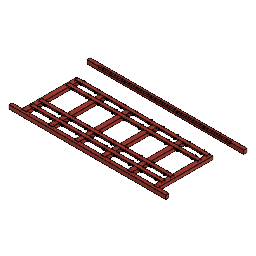
world (Autodesk Fusion 360 archive; units mm, degrees)
design "Maverick metal"
Autodesk Fusion 360 part; units mm, degrees
(part 1 of 2)
ref_plane "WorkPlane1" through (0, 0, -19.05) normal (0, 0, 1) x (1, 0, 0)
ref_plane "WorkPlane2" through (0, 0, -22.225) normal (0, 0, 1) x (1, 0, 0)
sketch "metal1" plane through (0, 0, 0) normal (0, 0, 1) x (1, 0, 0)
  circle A0 centre (67.0555, -55.245) radius 4.3815
  circle A1 centre (22.2245, -55.245) radius 4.3815
  circle A2 centre (25.2725, -93.218) radius 2.54
  circle A3 centre (64.0075, -93.218) radius 2.54
  line L0 (6.0955, -80.518) -> (-0.0005, -80.518)
  line L1 (6.0955, -96.393) -> (6.0955, -80.518)
  arc A4 (6.0955, -96.393) -> (9.2705, -99.568) centre (9.2705, -96.393) ccw
  line L2 (80.0095, -99.568) -> (9.2705, -99.568)
  arc A5 (80.0095, -99.568) -> (83.1845, -96.393) centre (80.0095, -96.393) ccw
  line L3 (83.1845, -80.518) -> (83.1845, -96.393)
  line L4 (89.2805, -80.518) -> (83.1845, -80.518)
  line L5 (89.2805, 938.276) -> (89.2805, -80.518)
  line L6 (-0.0005, 938.276) -> (89.2805, 938.276)
  line L7 (-0.0005, -80.518) -> (-0.0005, 938.276)
  circle A6 centre (2540.5075, -93.218) radius 2.54
  circle A7 centre (2543.5555, -55.245) radius 4.3815
  circle A8 centre (2498.7245, -55.245) radius 4.3815
  arc A9 (2501.7725, -95.758) -> (2501.7852, -90.678) centre (2501.7725, -93.218) ccw
  arc A10 (2501.7852, -90.678) -> (2501.7725, -95.758) centre (2501.7852, -93.218) ccw
  line L8 (2482.5955, -80.518) -> (2476.4995, -80.518)
  line L9 (2482.5955, -96.393) -> (2482.5955, -80.518)
  arc A11 (2482.5955, -96.393) -> (2485.7705, -99.568) centre (2485.7705, -96.393) ccw
  line L10 (2556.5095, -99.568) -> (2485.7705, -99.568)
  arc A12 (2556.5095, -99.568) -> (2559.6845, -96.393) centre (2556.5095, -96.393) ccw
  line L11 (2559.6845, -80.518) -> (2559.6845, -96.393)
  line L12 (2565.7805, -80.518) -> (2559.6845, -80.518)
  line L13 (2565.7805, 938.276) -> (2565.7805, -80.518)
  line L14 (2476.4995, 938.276) -> (2565.7805, 938.276)
  line L15 (2476.4995, -80.518) -> (2476.4995, 938.276)
  circle A13 centre (520.5725, -93.218) radius 2.54
  circle A14 centre (562.3555, -55.245) radius 4.3815
  circle A15 centre (517.5245, -55.245) radius 4.3815
  circle A16 centre (559.3075, -93.218) radius 2.54
  line L16 (501.3955, -80.518) -> (495.2995, -80.518)
  line L17 (501.3955, -96.393) -> (501.3955, -80.518)
  arc A17 (501.3955, -96.393) -> (504.5705, -99.568) centre (504.5705, -96.393) ccw
  line L18 (575.3095, -99.568) -> (504.5705, -99.568)
  arc A18 (575.3095, -99.568) -> (578.4845, -96.393) centre (575.3095, -96.393) ccw
  line L19 (578.4845, -80.518) -> (578.4845, -96.393)
  line L20 (584.5805, -80.518) -> (578.4845, -80.518)
  line L21 (584.5805, 938.276) -> (584.5805, -80.518)
  line L22 (495.2995, 938.276) -> (584.5805, 938.276)
  line L23 (495.2995, -80.518) -> (495.2995, 938.276)
  circle A19 centre (1549.9075, -93.218) radius 2.54
  circle A20 centre (1508.1245, -55.245) radius 4.3815
  circle A21 centre (1552.9555, -55.245) radius 4.3815
  arc A22 (1511.1852, -90.678) -> (1511.1725, -95.758) centre (1511.1852, -93.218) ccw
  arc A23 (1511.1725, -95.758) -> (1511.1852, -90.678) centre (1511.1725, -93.218) ccw
  line L24 (1491.9955, -80.518) -> (1485.8995, -80.518)
  line L25 (1491.9955, -96.393) -> (1491.9955, -80.518)
  arc A24 (1491.9955, -96.393) -> (1495.1705, -99.568) centre (1495.1705, -96.393) ccw
  line L26 (1565.9095, -99.568) -> (1495.1705, -99.568)
  arc A25 (1565.9095, -99.568) -> (1569.0845, -96.393) centre (1565.9095, -96.393) ccw
  line L27 (1569.0845, -80.518) -> (1569.0845, -96.393)
  line L28 (1575.1805, -80.518) -> (1569.0845, -80.518)
  line L29 (1575.1805, 938.276) -> (1575.1805, -80.518)
  line L30 (1485.8995, 938.276) -> (1575.1805, 938.276)
  line L31 (1485.8995, -80.518) -> (1485.8995, 938.276)
  circle A26 centre (2048.2555, -55.245) radius 4.3815
  circle A27 centre (2003.4245, -55.245) radius 4.3815
  arc A28 (2006.4725, -95.758) -> (2006.4852, -90.678) centre (2006.4725, -93.218) ccw
  arc A29 (2006.4852, -90.678) -> (2006.4725, -95.758) centre (2006.4852, -93.218) ccw
  arc A30 (2045.2075, -95.758) -> (2045.2202, -90.678) centre (2045.2075, -93.218) ccw
  arc A31 (2045.2202, -90.678) -> (2045.2075, -95.758) centre (2045.2202, -93.218) ccw
  line L32 (1987.2955, -80.518) -> (1981.1995, -80.518)
  line L33 (1987.2955, -96.393) -> (1987.2955, -80.518)
  arc A32 (1987.2955, -96.393) -> (1990.4705, -99.568) centre (1990.4705, -96.393) ccw
  line L34 (2061.2095, -99.568) -> (1990.4705, -99.568)
  arc A33 (2061.2095, -99.568) -> (2064.3845, -96.393) centre (2061.2095, -96.393) ccw
  line L35 (2064.3845, -80.518) -> (2064.3845, -96.393)
  line L36 (2070.4805, -80.518) -> (2064.3845, -80.518)
  line L37 (2070.4805, 938.276) -> (2070.4805, -80.518)
  line L38 (1981.1995, 938.276) -> (2070.4805, 938.276)
  line L39 (1981.1995, -80.518) -> (1981.1995, 938.276)
  circle A34 centre (1015.8725, -93.218) radius 2.54
  circle A35 centre (1012.8245, -55.245) radius 4.3815
  circle A36 centre (1057.6555, -55.245) radius 4.3815
  circle A37 centre (1054.6075, -93.218) radius 2.54
  line L40 (996.6955, -80.518) -> (990.5995, -80.518)
  line L41 (996.6955, -96.393) -> (996.6955, -80.518)
  arc A38 (996.6955, -96.393) -> (999.8705, -99.568) centre (999.8705, -96.393) ccw
  line L42 (1070.6095, -99.568) -> (999.8705, -99.568)
  arc A39 (1070.6095, -99.568) -> (1073.7845, -96.393) centre (1070.6095, -96.393) ccw
  line L43 (1073.7845, -80.518) -> (1073.7845, -96.393)
  line L44 (1079.8805, -80.518) -> (1073.7845, -80.518)
  line L45 (1079.8805, 938.276) -> (1079.8805, -80.518)
  line L46 (990.5995, 938.276) -> (1079.8805, 938.276)
  line L47 (990.5995, -80.518) -> (990.5995, 938.276)
sketch "metal2" plane through (0, 0, 0) normal (0, 0, 1) x (1, 0, 0)
  circle A0 centre (1690.5727, -112.268) radius 2.54
  circle A1 centre (1944.5727, -112.268) radius 2.54
  circle A2 centre (1891.2327, -112.268) radius 2.54
  circle A3 centre (621.2327, -112.268) radius 2.54
  circle A4 centre (2452.5727, -112.268) radius 2.54
  circle A5 centre (166.5727, -112.268) radius 2.54
  circle A6 centre (928.5727, -112.268) radius 2.54
  circle A7 centre (-87.4273, -112.268) radius 2.54
  circle A8 centre (1637.2327, -112.268) radius 2.54
  circle A9 centre (1436.5727, -112.268) radius 2.54
  circle A10 centre (367.2327, -112.268) radius 2.54
  circle A11 centre (1182.5727, -112.268) radius 2.54
  circle A12 centre (2145.2327, -112.268) radius 2.54
  circle A13 centre (2653.2327, -112.268) radius 2.54
  circle A14 centre (1383.2327, -112.268) radius 2.54
  circle A15 centre (420.5727, -112.268) radius 2.54
  circle A16 centre (875.2327, -112.268) radius 2.54
  circle A17 centre (2198.5727, -112.268) radius 2.54
  circle A18 centre (674.5727, -112.268) radius 2.54
  circle A19 centre (113.2327, -112.268) radius 2.54
  circle A20 centre (2399.2327, -112.268) radius 2.54
  circle A21 centre (1129.2327, -112.268) radius 2.54
  line L0 (2559.6845, -96.393) -> (2559.6845, -80.518)
  arc A22 (2556.5095, -99.568) -> (2559.6845, -96.393) centre (2556.5095, -96.393) ccw
  line L1 (2485.7705, -99.568) -> (2556.5095, -99.568)
  arc A23 (2482.5955, -96.393) -> (2485.7705, -99.568) centre (2485.7705, -96.393) ccw
  line L2 (2482.5955, -80.518) -> (2482.5955, -96.393)
  line L3 (2064.3845, -80.518) -> (2482.5955, -80.518)
  line L4 (2064.3845, -96.393) -> (2064.3845, -80.518)
  arc A24 (2061.2095, -99.568) -> (2064.3845, -96.393) centre (2061.2095, -96.393) ccw
  line L5 (1990.4705, -99.568) -> (2061.2095, -99.568)
  arc A25 (1987.2955, -96.393) -> (1990.4705, -99.568) centre (1990.4705, -96.393) ccw
  line L6 (1987.2955, -80.518) -> (1987.2955, -96.393)
  line L7 (1569.0845, -80.518) -> (1987.2955, -80.518)
  line L8 (1569.0845, -96.393) -> (1569.0845, -80.518)
  arc A26 (1565.9095, -99.568) -> (1569.0845, -96.393) centre (1565.9095, -96.393) ccw
  line L9 (1495.1705, -99.568) -> (1565.9095, -99.568)
  arc A27 (1491.9955, -96.393) -> (1495.1705, -99.568) centre (1495.1705, -96.393) ccw
  line L10 (1491.9955, -80.518) -> (1491.9955, -96.393)
  line L11 (1073.7845, -80.518) -> (1491.9955, -80.518)
  line L12 (1073.7845, -96.393) -> (1073.7845, -80.518)
  arc A28 (1070.6095, -99.568) -> (1073.7845, -96.393) centre (1070.6095, -96.393) ccw
  line L13 (999.8705, -99.568) -> (1070.6095, -99.568)
  arc A29 (996.6955, -96.393) -> (999.8705, -99.568) centre (999.8705, -96.393) ccw
  line L14 (996.6955, -80.518) -> (996.6955, -96.393)
  line L15 (578.4845, -80.518) -> (996.6955, -80.518)
  line L16 (578.4845, -96.393) -> (578.4845, -80.518)
  arc A30 (575.3095, -99.568) -> (578.4845, -96.393) centre (575.3095, -96.393) ccw
  line L17 (504.5705, -99.568) -> (575.3095, -99.568)
  arc A31 (501.3955, -96.393) -> (504.5705, -99.568) centre (504.5705, -96.393) ccw
  line L18 (501.3955, -80.518) -> (501.3955, -96.393)
  line L19 (83.1845, -80.518) -> (501.3955, -80.518)
  line L20 (83.1845, -96.393) -> (83.1845, -80.518)
  arc A32 (80.0095, -99.568) -> (83.1845, -96.393) centre (80.0095, -96.393) ccw
  line L21 (9.2705, -99.568) -> (80.0095, -99.568)
  arc A33 (6.0955, -96.393) -> (9.2705, -99.568) centre (9.2705, -96.393) ccw
  line L22 (6.0955, -80.518) -> (6.0955, -96.393)
  line L23 (-190.6783, -80.518) -> (6.0955, -80.518)
  line L24 (-190.6783, -144.018) -> (-190.6783, -80.518)
  line L25 (2756.4837, -144.018) -> (-190.6783, -144.018)
  line L26 (2756.4837, -80.518) -> (2756.4837, -144.018)
  line L27 (2559.6845, -80.518) -> (2756.4837, -80.518)
  circle A34 centre (1944.5727, 1354.074) radius 2.54
  circle A35 centre (1511.1979, 1335.024) radius 2.54
  circle A36 centre (1015.8725, 1335.024) radius 2.54
  circle A37 centre (1383.2327, 1354.074) radius 2.54
  circle A38 centre (2198.5727, 1354.074) radius 2.54
  circle A39 centre (2540.5329, 1335.024) radius 2.54
  circle A40 centre (2399.2327, 1354.074) radius 2.54
  circle A41 centre (2006.4979, 1335.024) radius 2.54
  circle A42 centre (1549.9329, 1335.024) radius 2.54
  circle A43 centre (1891.2327, 1354.074) radius 2.54
  circle A44 centre (2045.2329, 1335.024) radius 2.54
  circle A45 centre (674.5727, 1354.074) radius 2.54
  circle A46 centre (875.2327, 1354.074) radius 2.54
  circle A47 centre (367.2327, 1354.074) radius 2.54
  circle A48 centre (621.2327, 1354.074) radius 2.54
  circle A49 centre (520.5725, 1335.024) radius 2.54
  circle A50 centre (-87.4273, 1354.074) radius 2.54
  circle A51 centre (166.5727, 1354.074) radius 2.54
  circle A52 centre (1436.5727, 1354.074) radius 2.54
  circle A53 centre (2501.7979, 1335.024) radius 2.54
  circle A54 centre (1690.5727, 1354.074) radius 2.54
  circle A55 centre (928.5727, 1354.074) radius 2.54
  circle A56 centre (1637.2327, 1354.074) radius 2.54
  circle A57 centre (2653.2327, 1354.074) radius 2.54
  circle A58 centre (1054.6075, 1335.024) radius 2.54
  circle A59 centre (2145.2327, 1354.074) radius 2.54
  circle A60 centre (1182.5727, 1354.074) radius 2.54
  circle A61 centre (559.3075, 1335.024) radius 2.54
  circle A62 centre (2452.5727, 1354.074) radius 2.54
  circle A63 centre (113.2327, 1354.074) radius 2.54
  circle A64 centre (25.2725, 1335.024) radius 2.54
  circle A65 centre (1129.2327, 1354.074) radius 2.54
  circle A66 centre (64.0075, 1335.024) radius 2.54
  circle A67 centre (420.5727, 1354.074) radius 2.54
  line L28 (-190.6783, 1322.324) -> (-190.6783, 1385.824)
  line L29 (2756.4837, 1322.324) -> (-190.6783, 1322.324)
  line L30 (2756.4837, 1385.824) -> (2756.4837, 1322.324)
  line L31 (-190.6783, 1385.824) -> (2756.4837, 1385.824)
sketch "metal0" plane through (0, 0, 0) normal (0, 0, 1) x (1, 0, 0)
  circle A0 centre (1282.5725, 1306.576) radius 4.3815
  line L0 (1035.5575, 1322.324) -> (1529.5875, 1322.324)
  line L1 (1035.5575, 1303.274) -> (1035.5575, 1322.324)
  arc A1 (1035.5575, 1303.274) -> (1041.9075, 1296.924) centre (1041.9075, 1303.274) ccw
  line L2 (1523.2375, 1296.924) -> (1041.9075, 1296.924)
  arc A2 (1523.2375, 1296.924) -> (1529.5875, 1303.274) centre (1523.2375, 1303.274) ccw
  line L3 (1529.5875, 1322.324) -> (1529.5875, 1303.274)
  circle A3 centre (2273.1725, 1306.576) radius 4.3815
  line L4 (2026.1575, 1322.324) -> (2520.1875, 1322.324)
  line L5 (2026.1575, 1303.274) -> (2026.1575, 1322.324)
  arc A4 (2026.1575, 1303.274) -> (2032.5075, 1296.924) centre (2032.5075, 1303.274) ccw
  line L6 (2513.8375, 1296.924) -> (2032.5075, 1296.924)
  arc A5 (2513.8375, 1296.924) -> (2520.1875, 1303.274) centre (2513.8375, 1303.274) ccw
  line L7 (2520.1875, 1322.324) -> (2520.1875, 1303.274)
  circle A6 centre (1777.8725, 1306.576) radius 4.3815
  line L8 (1530.8575, 1303.274) -> (1530.8575, 1322.324)
  arc A7 (1530.8575, 1303.274) -> (1537.2075, 1296.924) centre (1537.2075, 1303.274) ccw
  line L9 (2018.5375, 1296.924) -> (1537.2075, 1296.924)
  arc A8 (2018.5375, 1296.924) -> (2024.8875, 1303.274) centre (2018.5375, 1303.274) ccw
  line L10 (2024.8875, 1322.324) -> (2024.8875, 1303.274)
  line L11 (1530.8575, 1322.324) -> (2024.8875, 1322.324)
  circle A9 centre (291.9725, 1306.576) radius 4.3815
  line L12 (44.9575, 1303.274) -> (44.9575, 1322.324)
  arc A10 (44.9575, 1303.274) -> (51.3075, 1296.924) centre (51.3075, 1303.274) ccw
  line L13 (532.6375, 1296.924) -> (51.3075, 1296.924)
  arc A11 (532.6375, 1296.924) -> (538.9875, 1303.274) centre (532.6375, 1303.274) ccw
  line L14 (538.9875, 1322.324) -> (538.9875, 1303.274)
  line L15 (44.9575, 1322.324) -> (538.9875, 1322.324)
  circle A12 centre (787.2725, 1306.576) radius 4.3815
  line L16 (540.2575, 1322.324) -> (1034.2875, 1322.324)
  line L17 (540.2575, 1303.274) -> (540.2575, 1322.324)
  arc A13 (540.2575, 1303.274) -> (546.6075, 1296.924) centre (546.6075, 1303.274) ccw
  line L18 (1027.9375, 1296.924) -> (546.6075, 1296.924)
  arc A14 (1027.9375, 1296.924) -> (1034.2875, 1303.274) centre (1027.9375, 1303.274) ccw
  line L19 (1034.2875, 1322.324) -> (1034.2875, 1303.274)
  circle A15 centre (2410.2055, 86.1695) radius 4.3815
  circle A16 centre (429.0055, 9.9695) radius 4.3815
  circle A17 centre (1641.8555, 9.9695) radius 4.3815
  circle A18 centre (651.2555, 9.9695) radius 4.3815
  circle A19 centre (1914.9055, 9.9695) radius 4.3815
  circle A20 centre (1146.5555, 86.1695) radius 4.3815
  circle A21 centre (429.0055, 86.1695) radius 4.3815
  circle A22 centre (1641.8555, 86.1695) radius 4.3815
  circle A23 centre (155.9555, 9.9695) radius 4.3815
  circle A24 centre (155.9555, 86.1695) radius 4.3815
  circle A25 centre (2137.1555, 9.9695) radius 4.3815
  circle A26 centre (1419.6055, 86.1695) radius 4.3815
  circle A27 centre (2137.1555, 86.1695) radius 4.3815
  circle A28 centre (651.2555, 86.1695) radius 4.3815
  circle A29 centre (924.3055, 9.9695) radius 4.3815
  circle A30 centre (2410.2055, 9.9695) radius 4.3815
  circle A31 centre (1146.5555, 9.9695) radius 4.3815
  circle A32 centre (924.3055, 86.1695) radius 4.3815
  circle A33 centre (1419.6055, 9.9695) radius 4.3815
  circle A34 centre (1914.9055, 86.1695) radius 4.3815
  line L20 (2432.4305, 79.8195) -> (2521.3305, 79.8195)
  line L21 (2432.4305, 71.8185) -> (2432.4305, 79.8195)
  arc A35 (2430.9065, 70.2945) -> (2432.4305, 71.8185) centre (2430.9065, 71.8185) ccw
  line L22 (2427.6045, 70.2945) -> (2430.9065, 70.2945)
  arc A36 (2426.0805, 71.8185) -> (2427.6045, 70.2945) centre (2427.6045, 71.8185) ccw
  line L23 (2426.0805, 86.1695) -> (2426.0805, 71.8185)
  arc A37 (2426.0805, 86.1695) -> (2416.5555, 95.6945) centre (2416.5555, 86.1695) ccw
  line L24 (2403.8555, 95.6945) -> (2416.5555, 95.6945)
  arc A38 (2403.8555, 95.6945) -> (2394.3305, 86.1695) centre (2403.8555, 86.1695) ccw
  line L25 (2394.3305, 71.8185) -> (2394.3305, 86.1695)
  arc A39 (2392.8065, 70.2945) -> (2394.3305, 71.8185) centre (2392.8065, 71.8185) ccw
  line L26 (2389.5045, 70.2945) -> (2392.8065, 70.2945)
  arc A40 (2387.9805, 71.8185) -> (2389.5045, 70.2945) centre (2389.5045, 71.8185) ccw
  line L27 (2387.9805, 79.8195) -> (2387.9805, 71.8185)
  line L28 (2159.3805, 79.8195) -> (2387.9805, 79.8195)
  line L29 (2159.3805, 71.8185) -> (2159.3805, 79.8195)
  arc A41 (2157.8565, 70.2945) -> (2159.3805, 71.8185) centre (2157.8565, 71.8185) ccw
  line L30 (2154.5545, 70.2945) -> (2157.8565, 70.2945)
  arc A42 (2153.0305, 71.8185) -> (2154.5545, 70.2945) centre (2154.5545, 71.8185) ccw
  line L31 (2153.0305, 86.1695) -> (2153.0305, 71.8185)
  arc A43 (2153.0305, 86.1695) -> (2143.5055, 95.6945) centre (2143.5055, 86.1695) ccw
  line L32 (2130.8055, 95.6945) -> (2143.5055, 95.6945)
  arc A44 (2130.8055, 95.6945) -> (2121.2805, 86.1695) centre (2130.8055, 86.1695) ccw
  line L33 (2121.2805, 71.8185) -> (2121.2805, 86.1695)
  arc A45 (2119.7565, 70.2945) -> (2121.2805, 71.8185) centre (2119.7565, 71.8185) ccw
  line L34 (2116.4545, 70.2945) -> (2119.7565, 70.2945)
  arc A46 (2114.9305, 71.8185) -> (2116.4545, 70.2945) centre (2116.4545, 71.8185) ccw
  line L35 (2114.9305, 79.8195) -> (2114.9305, 71.8185)
  line L36 (1937.1305, 79.8195) -> (2114.9305, 79.8195)
  line L37 (1937.1305, 71.8185) -> (1937.1305, 79.8195)
  arc A47 (1935.6065, 70.2945) -> (1937.1305, 71.8185) centre (1935.6065, 71.8185) ccw
  line L38 (1932.3045, 70.2945) -> (1935.6065, 70.2945)
  arc A48 (1930.7805, 71.8185) -> (1932.3045, 70.2945) centre (1932.3045, 71.8185) ccw
  line L39 (1930.7805, 86.1695) -> (1930.7805, 71.8185)
  arc A49 (1930.7805, 86.1695) -> (1921.2555, 95.6945) centre (1921.2555, 86.1695) ccw
  line L40 (1908.5555, 95.6945) -> (1921.2555, 95.6945)
  arc A50 (1908.5555, 95.6945) -> (1899.0305, 86.1695) centre (1908.5555, 86.1695) ccw
  line L41 (1899.0305, 71.8185) -> (1899.0305, 86.1695)
  arc A51 (1897.5065, 70.2945) -> (1899.0305, 71.8185) centre (1897.5065, 71.8185) ccw
  line L42 (1894.2045, 70.2945) -> (1897.5065, 70.2945)
  arc A52 (1892.6805, 71.8185) -> (1894.2045, 70.2945) centre (1894.2045, 71.8185) ccw
  line L43 (1892.6805, 79.8195) -> (1892.6805, 71.8185)
  line L44 (1664.0805, 79.8195) -> (1892.6805, 79.8195)
  line L45 (1664.0805, 71.8185) -> (1664.0805, 79.8195)
  arc A53 (1662.5565, 70.2945) -> (1664.0805, 71.8185) centre (1662.5565, 71.8185) ccw
  line L46 (1659.2545, 70.2945) -> (1662.5565, 70.2945)
  arc A54 (1657.7305, 71.8185) -> (1659.2545, 70.2945) centre (1659.2545, 71.8185) ccw
  line L47 (1657.7305, 86.1695) -> (1657.7305, 71.8185)
  arc A55 (1657.7305, 86.1695) -> (1648.2055, 95.6945) centre (1648.2055, 86.1695) ccw
  line L48 (1635.5055, 95.6945) -> (1648.2055, 95.6945)
  arc A56 (1635.5055, 95.6945) -> (1625.9805, 86.1695) centre (1635.5055, 86.1695) ccw
  line L49 (1625.9805, 71.8185) -> (1625.9805, 86.1695)
  arc A57 (1624.4565, 70.2945) -> (1625.9805, 71.8185) centre (1624.4565, 71.8185) ccw
  line L50 (1621.1545, 70.2945) -> (1624.4565, 70.2945)
  arc A58 (1619.6305, 71.8185) -> (1621.1545, 70.2945) centre (1621.1545, 71.8185) ccw
  line L51 (1619.6305, 79.8195) -> (1619.6305, 71.8185)
  line L52 (1441.8305, 79.8195) -> (1619.6305, 79.8195)
  line L53 (1441.8305, 71.8185) -> (1441.8305, 79.8195)
  arc A59 (1440.3065, 70.2945) -> (1441.8305, 71.8185) centre (1440.3065, 71.8185) ccw
  line L54 (1437.0045, 70.2945) -> (1440.3065, 70.2945)
  arc A60 (1435.4805, 71.8185) -> (1437.0045, 70.2945) centre (1437.0045, 71.8185) ccw
  line L55 (1435.4805, 86.1695) -> (1435.4805, 71.8185)
  arc A61 (1435.4805, 86.1695) -> (1425.9555, 95.6945) centre (1425.9555, 86.1695) ccw
  line L56 (1413.2555, 95.6945) -> (1425.9555, 95.6945)
  arc A62 (1413.2555, 95.6945) -> (1403.7305, 86.1695) centre (1413.2555, 86.1695) ccw
  line L57 (1403.7305, 71.8185) -> (1403.7305, 86.1695)
  arc A63 (1402.2065, 70.2945) -> (1403.7305, 71.8185) centre (1402.2065, 71.8185) ccw
  line L58 (1398.9045, 70.2945) -> (1402.2065, 70.2945)
  arc A64 (1397.3805, 71.8185) -> (1398.9045, 70.2945) centre (1398.9045, 71.8185) ccw
  line L59 (1397.3805, 79.8195) -> (1397.3805, 71.8185)
  line L60 (1168.7805, 79.8195) -> (1397.3805, 79.8195)
  line L61 (1168.7805, 71.8185) -> (1168.7805, 79.8195)
  arc A65 (1167.2565, 70.2945) -> (1168.7805, 71.8185) centre (1167.2565, 71.8185) ccw
  line L62 (1163.9545, 70.2945) -> (1167.2565, 70.2945)
  arc A66 (1162.4305, 71.8185) -> (1163.9545, 70.2945) centre (1163.9545, 71.8185) ccw
  line L63 (1162.4305, 86.1695) -> (1162.4305, 71.8185)
  arc A67 (1162.4305, 86.1695) -> (1152.9055, 95.6945) centre (1152.9055, 86.1695) ccw
  line L64 (1140.2055, 95.6945) -> (1152.9055, 95.6945)
  arc A68 (1140.2055, 95.6945) -> (1130.6805, 86.1695) centre (1140.2055, 86.1695) ccw
  line L65 (1130.6805, 71.8185) -> (1130.6805, 86.1695)
  arc A69 (1129.1565, 70.2945) -> (1130.6805, 71.8185) centre (1129.1565, 71.8185) ccw
  line L66 (1125.8545, 70.2945) -> (1129.1565, 70.2945)
  arc A70 (1124.3305, 71.8185) -> (1125.8545, 70.2945) centre (1125.8545, 71.8185) ccw
  line L67 (1124.3305, 79.8195) -> (1124.3305, 71.8185)
  line L68 (946.5305, 79.8195) -> (1124.3305, 79.8195)
  line L69 (946.5305, 71.8185) -> (946.5305, 79.8195)
  arc A71 (945.0065, 70.2945) -> (946.5305, 71.8185) centre (945.0065, 71.8185) ccw
  line L70 (941.7045, 70.2945) -> (945.0065, 70.2945)
  arc A72 (940.1805, 71.8185) -> (941.7045, 70.2945) centre (941.7045, 71.8185) ccw
  line L71 (940.1805, 86.1695) -> (940.1805, 71.8185)
  arc A73 (940.1805, 86.1695) -> (930.6555, 95.6945) centre (930.6555, 86.1695) ccw
  line L72 (917.9555, 95.6945) -> (930.6555, 95.6945)
  arc A74 (917.9555, 95.6945) -> (908.4305, 86.1695) centre (917.9555, 86.1695) ccw
  line L73 (908.4305, 71.8185) -> (908.4305, 86.1695)
  arc A75 (906.9065, 70.2945) -> (908.4305, 71.8185) centre (906.9065, 71.8185) ccw
  line L74 (903.6045, 70.2945) -> (906.9065, 70.2945)
  arc A76 (902.0805, 71.8185) -> (903.6045, 70.2945) centre (903.6045, 71.8185) ccw
  line L75 (902.0805, 79.8195) -> (902.0805, 71.8185)
  line L76 (673.4805, 79.8195) -> (902.0805, 79.8195)
  line L77 (673.4805, 71.8185) -> (673.4805, 79.8195)
  arc A77 (671.9565, 70.2945) -> (673.4805, 71.8185) centre (671.9565, 71.8185) ccw
  line L78 (668.6545, 70.2945) -> (671.9565, 70.2945)
  arc A78 (667.1305, 71.8185) -> (668.6545, 70.2945) centre (668.6545, 71.8185) ccw
  line L79 (667.1305, 86.1695) -> (667.1305, 71.8185)
  arc A79 (667.1305, 86.1695) -> (657.6055, 95.6945) centre (657.6055, 86.1695) ccw
  line L80 (644.9055, 95.6945) -> (657.6055, 95.6945)
  arc A80 (644.9055, 95.6945) -> (635.3805, 86.1695) centre (644.9055, 86.1695) ccw
  line L81 (635.3805, 71.8185) -> (635.3805, 86.1695)
  arc A81 (633.8565, 70.2945) -> (635.3805, 71.8185) centre (633.8565, 71.8185) ccw
  line L82 (630.5545, 70.2945) -> (633.8565, 70.2945)
  arc A82 (629.0305, 71.8185) -> (630.5545, 70.2945) centre (630.5545, 71.8185) ccw
  line L83 (629.0305, 79.8195) -> (629.0305, 71.8185)
  line L84 (451.2305, 79.8195) -> (629.0305, 79.8195)
  line L85 (451.2305, 71.8185) -> (451.2305, 79.8195)
  arc A83 (449.7065, 70.2945) -> (451.2305, 71.8185) centre (449.7065, 71.8185) ccw
  line L86 (446.4045, 70.2945) -> (449.7065, 70.2945)
  arc A84 (444.8805, 71.8185) -> (446.4045, 70.2945) centre (446.4045, 71.8185) ccw
  line L87 (444.8805, 86.1695) -> (444.8805, 71.8185)
  arc A85 (444.8805, 86.1695) -> (435.3555, 95.6945) centre (435.3555, 86.1695) ccw
  line L88 (422.6555, 95.6945) -> (435.3555, 95.6945)
  arc A86 (422.6555, 95.6945) -> (413.1305, 86.1695) centre (422.6555, 86.1695) ccw
  line L89 (413.1305, 71.8185) -> (413.1305, 86.1695)
  arc A87 (411.6065, 70.2945) -> (413.1305, 71.8185) centre (411.6065, 71.8185) ccw
  line L90 (408.3045, 70.2945) -> (411.6065, 70.2945)
  arc A88 (406.7805, 71.8185) -> (408.3045, 70.2945) centre (408.3045, 71.8185) ccw
  line L91 (406.7805, 79.8195) -> (406.7805, 71.8185)
  line L92 (178.1805, 79.8195) -> (406.7805, 79.8195)
  line L93 (178.1805, 71.8185) -> (178.1805, 79.8195)
  arc A89 (176.6565, 70.2945) -> (178.1805, 71.8185) centre (176.6565, 71.8185) ccw
  line L94 (173.3545, 70.2945) -> (176.6565, 70.2945)
  arc A90 (171.8305, 71.8185) -> (173.3545, 70.2945) centre (173.3545, 71.8185) ccw
  line L95 (171.8305, 86.1695) -> (171.8305, 71.8185)
  arc A91 (171.8305, 86.1695) -> (162.3055, 95.6945) centre (162.3055, 86.1695) ccw
  line L96 (149.6055, 95.6945) -> (162.3055, 95.6945)
  arc A92 (149.6055, 95.6945) -> (140.0805, 86.1695) centre (149.6055, 86.1695) ccw
  line L97 (140.0805, 71.8185) -> (140.0805, 86.1695)
  arc A93 (138.5565, 70.2945) -> (140.0805, 71.8185) centre (138.5565, 71.8185) ccw
  line L98 (135.2545, 70.2945) -> (138.5565, 70.2945)
  arc A94 (133.7305, 71.8185) -> (135.2545, 70.2945) centre (135.2545, 71.8185) ccw
  line L99 (133.7305, 79.8195) -> (133.7305, 71.8185)
  line L100 (44.8305, 79.8195) -> (133.7305, 79.8195)
  line L101 (44.8305, 16.3195) -> (44.8305, 79.8195)
  line L102 (133.7305, 16.3195) -> (44.8305, 16.3195)
  line L103 (133.7305, 24.3205) -> (133.7305, 16.3195)
  arc A95 (135.2545, 25.8445) -> (133.7305, 24.3205) centre (135.2545, 24.3205) ccw
  line L104 (138.5565, 25.8445) -> (135.2545, 25.8445)
  arc A96 (140.0805, 24.3205) -> (138.5565, 25.8445) centre (138.5565, 24.3205) ccw
  line L105 (140.0805, 9.9695) -> (140.0805, 24.3205)
  arc A97 (140.0805, 9.9695) -> (149.6055, 0.4445) centre (149.6055, 9.9695) ccw
  line L106 (162.3055, 0.4445) -> (149.6055, 0.4445)
  arc A98 (162.3055, 0.4445) -> (171.8305, 9.9695) centre (162.3055, 9.9695) ccw
  line L107 (171.8305, 24.3205) -> (171.8305, 9.9695)
  arc A99 (173.3545, 25.8445) -> (171.8305, 24.3205) centre (173.3545, 24.3205) ccw
  line L108 (176.6565, 25.8445) -> (173.3545, 25.8445)
  arc A100 (178.1805, 24.3205) -> (176.6565, 25.8445) centre (176.6565, 24.3205) ccw
  line L109 (178.1805, 16.3195) -> (178.1805, 24.3205)
  line L110 (406.7805, 16.3195) -> (178.1805, 16.3195)
  line L111 (406.7805, 24.3205) -> (406.7805, 16.3195)
  arc A101 (408.3045, 25.8445) -> (406.7805, 24.3205) centre (408.3045, 24.3205) ccw
  line L112 (411.6065, 25.8445) -> (408.3045, 25.8445)
  arc A102 (413.1305, 24.3205) -> (411.6065, 25.8445) centre (411.6065, 24.3205) ccw
  line L113 (413.1305, 9.9695) -> (413.1305, 24.3205)
  arc A103 (413.1305, 9.9695) -> (422.6555, 0.4445) centre (422.6555, 9.9695) ccw
  line L114 (435.3555, 0.4445) -> (422.6555, 0.4445)
  arc A104 (435.3555, 0.4445) -> (444.8805, 9.9695) centre (435.3555, 9.9695) ccw
  line L115 (444.8805, 24.3205) -> (444.8805, 9.9695)
  arc A105 (446.4045, 25.8445) -> (444.8805, 24.3205) centre (446.4045, 24.3205) ccw
  line L116 (449.7065, 25.8445) -> (446.4045, 25.8445)
  arc A106 (451.2305, 24.3205) -> (449.7065, 25.8445) centre (449.7065, 24.3205) ccw
  line L117 (451.2305, 16.3195) -> (451.2305, 24.3205)
  line L118 (629.0305, 16.3195) -> (451.2305, 16.3195)
  line L119 (629.0305, 24.3205) -> (629.0305, 16.3195)
  arc A107 (630.5545, 25.8445) -> (629.0305, 24.3205) centre (630.5545, 24.3205) ccw
  line L120 (633.8565, 25.8445) -> (630.5545, 25.8445)
  arc A108 (635.3805, 24.3205) -> (633.8565, 25.8445) centre (633.8565, 24.3205) ccw
  line L121 (635.3805, 9.9695) -> (635.3805, 24.3205)
  arc A109 (635.3805, 9.9695) -> (644.9055, 0.4445) centre (644.9055, 9.9695) ccw
  line L122 (657.6055, 0.4445) -> (644.9055, 0.4445)
  arc A110 (657.6055, 0.4445) -> (667.1305, 9.9695) centre (657.6055, 9.9695) ccw
  line L123 (667.1305, 24.3205) -> (667.1305, 9.9695)
  arc A111 (668.6545, 25.8445) -> (667.1305, 24.3205) centre (668.6545, 24.3205) ccw
  line L124 (671.9565, 25.8445) -> (668.6545, 25.8445)
  arc A112 (673.4805, 24.3205) -> (671.9565, 25.8445) centre (671.9565, 24.3205) ccw
  line L125 (673.4805, 16.3195) -> (673.4805, 24.3205)
  line L126 (902.0805, 16.3195) -> (673.4805, 16.3195)
  line L127 (902.0805, 24.3205) -> (902.0805, 16.3195)
  arc A113 (903.6045, 25.8445) -> (902.0805, 24.3205) centre (903.6045, 24.3205) ccw
  line L128 (906.9065, 25.8445) -> (903.6045, 25.8445)
  arc A114 (908.4305, 24.3205) -> (906.9065, 25.8445) centre (906.9065, 24.3205) ccw
  line L129 (908.4305, 9.9695) -> (908.4305, 24.3205)
  arc A115 (908.4305, 9.9695) -> (917.9555, 0.4445) centre (917.9555, 9.9695) ccw
  line L130 (930.6555, 0.4445) -> (917.9555, 0.4445)
  arc A116 (930.6555, 0.4445) -> (940.1805, 9.9695) centre (930.6555, 9.9695) ccw
  line L131 (940.1805, 24.3205) -> (940.1805, 9.9695)
  arc A117 (941.7045, 25.8445) -> (940.1805, 24.3205) centre (941.7045, 24.3205) ccw
  line L132 (945.0065, 25.8445) -> (941.7045, 25.8445)
  arc A118 (946.5305, 24.3205) -> (945.0065, 25.8445) centre (945.0065, 24.3205) ccw
  line L133 (946.5305, 16.3195) -> (946.5305, 24.3205)
  line L134 (1124.3305, 16.3195) -> (946.5305, 16.3195)
  line L135 (1124.3305, 24.3205) -> (1124.3305, 16.3195)
  arc A119 (1125.8545, 25.8445) -> (1124.3305, 24.3205) centre (1125.8545, 24.3205) ccw
  line L136 (1129.1565, 25.8445) -> (1125.8545, 25.8445)
  arc A120 (1130.6805, 24.3205) -> (1129.1565, 25.8445) centre (1129.1565, 24.3205) ccw
  line L137 (1130.6805, 9.9695) -> (1130.6805, 24.3205)
  arc A121 (1130.6805, 9.9695) -> (1140.2055, 0.4445) centre (1140.2055, 9.9695) ccw
  line L138 (1152.9055, 0.4445) -> (1140.2055, 0.4445)
  arc A122 (1152.9055, 0.4445) -> (1162.4305, 9.9695) centre (1152.9055, 9.9695) ccw
  line L139 (1162.4305, 24.3205) -> (1162.4305, 9.9695)
  arc A123 (1163.9545, 25.8445) -> (1162.4305, 24.3205) centre (1163.9545, 24.3205) ccw
  line L140 (1167.2565, 25.8445) -> (1163.9545, 25.8445)
  arc A124 (1168.7805, 24.3205) -> (1167.2565, 25.8445) centre (1167.2565, 24.3205) ccw
  line L141 (1168.7805, 16.3195) -> (1168.7805, 24.3205)
  line L142 (1397.3805, 16.3195) -> (1168.7805, 16.3195)
  line L143 (1397.3805, 24.3205) -> (1397.3805, 16.3195)
  arc A125 (1398.9045, 25.8445) -> (1397.3805, 24.3205) centre (1398.9045, 24.3205) ccw
  line L144 (1402.2065, 25.8445) -> (1398.9045, 25.8445)
  arc A126 (1403.7305, 24.3205) -> (1402.2065, 25.8445) centre (1402.2065, 24.3205) ccw
  line L145 (1403.7305, 9.9695) -> (1403.7305, 24.3205)
  arc A127 (1403.7305, 9.9695) -> (1413.2555, 0.4445) centre (1413.2555, 9.9695) ccw
  line L146 (1425.9555, 0.4445) -> (1413.2555, 0.4445)
  arc A128 (1425.9555, 0.4445) -> (1435.4805, 9.9695) centre (1425.9555, 9.9695) ccw
  line L147 (1435.4805, 24.3205) -> (1435.4805, 9.9695)
  arc A129 (1437.0045, 25.8445) -> (1435.4805, 24.3205) centre (1437.0045, 24.3205) ccw
  line L148 (1440.3065, 25.8445) -> (1437.0045, 25.8445)
  arc A130 (1441.8305, 24.3205) -> (1440.3065, 25.8445) centre (1440.3065, 24.3205) ccw
  line L149 (1441.8305, 16.3195) -> (1441.8305, 24.3205)
  line L150 (1619.6305, 16.3195) -> (1441.8305, 16.3195)
  line L151 (1619.6305, 24.3205) -> (1619.6305, 16.3195)
  arc A131 (1621.1545, 25.8445) -> (1619.6305, 24.3205) centre (1621.1545, 24.3205) ccw
  line L152 (1624.4565, 25.8445) -> (1621.1545, 25.8445)
  arc A132 (1625.9805, 24.3205) -> (1624.4565, 25.8445) centre (1624.4565, 24.3205) ccw
  line L153 (1625.9805, 9.9695) -> (1625.9805, 24.3205)
  arc A133 (1625.9805, 9.9695) -> (1635.5055, 0.4445) centre (1635.5055, 9.9695) ccw
  line L154 (1648.2055, 0.4445) -> (1635.5055, 0.4445)
  arc A134 (1648.2055, 0.4445) -> (1657.7305, 9.9695) centre (1648.2055, 9.9695) ccw
  line L155 (1657.7305, 24.3205) -> (1657.7305, 9.9695)
  arc A135 (1659.2545, 25.8445) -> (1657.7305, 24.3205) centre (1659.2545, 24.3205) ccw
  line L156 (1662.5565, 25.8445) -> (1659.2545, 25.8445)
  arc A136 (1664.0805, 24.3205) -> (1662.5565, 25.8445) centre (1662.5565, 24.3205) ccw
  line L157 (1664.0805, 16.3195) -> (1664.0805, 24.3205)
  line L158 (1892.6805, 16.3195) -> (1664.0805, 16.3195)
  line L159 (1892.6805, 24.3205) -> (1892.6805, 16.3195)
  arc A137 (1894.2045, 25.8445) -> (1892.6805, 24.3205) centre (1894.2045, 24.3205) ccw
  line L160 (1897.5065, 25.8445) -> (1894.2045, 25.8445)
  arc A138 (1899.0305, 24.3205) -> (1897.5065, 25.8445) centre (1897.5065, 24.3205) ccw
  line L161 (1899.0305, 9.9695) -> (1899.0305, 24.3205)
  arc A139 (1899.0305, 9.9695) -> (1908.5555, 0.4445) centre (1908.5555, 9.9695) ccw
  line L162 (1921.2555, 0.4445) -> (1908.5555, 0.4445)
  arc A140 (1921.2555, 0.4445) -> (1930.7805, 9.9695) centre (1921.2555, 9.9695) ccw
  line L163 (1930.7805, 24.3205) -> (1930.7805, 9.9695)
  arc A141 (1932.3045, 25.8445) -> (1930.7805, 24.3205) centre (1932.3045, 24.3205) ccw
  line L164 (1935.6065, 25.8445) -> (1932.3045, 25.8445)
  arc A142 (1937.1305, 24.3205) -> (1935.6065, 25.8445) centre (1935.6065, 24.3205) ccw
  line L165 (1937.1305, 16.3195) -> (1937.1305, 24.3205)
  line L166 (2114.9305, 16.3195) -> (1937.1305, 16.3195)
  line L167 (2114.9305, 24.3205) -> (2114.9305, 16.3195)
  arc A143 (2116.4545, 25.8445) -> (2114.9305, 24.3205) centre (2116.4545, 24.3205) ccw
  line L168 (2119.7565, 25.8445) -> (2116.4545, 25.8445)
  arc A144 (2121.2805, 24.3205) -> (2119.7565, 25.8445) centre (2119.7565, 24.3205) ccw
  line L169 (2121.2805, 9.9695) -> (2121.2805, 24.3205)
  arc A145 (2121.2805, 9.9695) -> (2130.8055, 0.4445) centre (2130.8055, 9.9695) ccw
  line L170 (2143.5055, 0.4445) -> (2130.8055, 0.4445)
  arc A146 (2143.5055, 0.4445) -> (2153.0305, 9.9695) centre (2143.5055, 9.9695) ccw
  line L171 (2153.0305, 24.3205) -> (2153.0305, 9.9695)
  arc A147 (2154.5545, 25.8445) -> (2153.0305, 24.3205) centre (2154.5545, 24.3205) ccw
  line L172 (2157.8565, 25.8445) -> (2154.5545, 25.8445)
  arc A148 (2159.3805, 24.3205) -> (2157.8565, 25.8445) centre (2157.8565, 24.3205) ccw
  line L173 (2159.3805, 16.3195) -> (2159.3805, 24.3205)
  line L174 (2387.9805, 16.3195) -> (2159.3805, 16.3195)
  line L175 (2387.9805, 24.3205) -> (2387.9805, 16.3195)
  arc A149 (2389.5045, 25.8445) -> (2387.9805, 24.3205) centre (2389.5045, 24.3205) ccw
  line L176 (2392.8065, 25.8445) -> (2389.5045, 25.8445)
  arc A150 (2394.3305, 24.3205) -> (2392.8065, 25.8445) centre (2392.8065, 24.3205) ccw
  line L177 (2394.3305, 9.9695) -> (2394.3305, 24.3205)
  arc A151 (2394.3305, 9.9695) -> (2403.8555, 0.4445) centre (2403.8555, 9.9695) ccw
  line L178 (2416.5555, 0.4445) -> (2403.8555, 0.4445)
  arc A152 (2416.5555, 0.4445) -> (2426.0805, 9.9695) centre (2416.5555, 9.9695) ccw
  line L179 (2426.0805, 24.3205) -> (2426.0805, 9.9695)
  arc A153 (2427.6045, 25.8445) -> (2426.0805, 24.3205) centre (2427.6045, 24.3205) ccw
  line L180 (2430.9065, 25.8445) -> (2427.6045, 25.8445)
  arc A154 (2432.4305, 24.3205) -> (2430.9065, 25.8445) centre (2430.9065, 24.3205) ccw
  line L181 (2432.4305, 16.3195) -> (2432.4305, 24.3205)
  line L182 (2521.3305, 16.3195) -> (2432.4305, 16.3195)
  line L183 (2521.3305, 79.8195) -> (2521.3305, 16.3195)
  line L184 (1167.2565, 190.9445) -> (1163.9545, 190.9445)
  line L185 (1162.4305, 251.2695) -> (1162.4305, 236.9185)
  circle A155 centre (2137.1555, 251.2695) radius 4.3815
  arc A156 (2143.5055, 165.5445) -> (2153.0305, 175.0695) centre (2143.5055, 175.0695) ccw
  line L186 (1163.9545, 235.3945) -> (1167.2565, 235.3945)
  line L187 (2154.5545, 235.3945) -> (2157.8565, 235.3945)
  line L188 (2387.9805, 181.4195) -> (2159.3805, 181.4195)
  arc A157 (2119.7565, 235.3945) -> (2121.2805, 236.9185) centre (2119.7565, 236.9185) ccw
  arc A158 (2159.3805, 189.4205) -> (2157.8565, 190.9445) centre (2157.8565, 189.4205) ccw
  arc A159 (633.8565, 235.3945) -> (635.3805, 236.9185) centre (633.8565, 236.9185) ccw
  line L189 (2157.8565, 190.9445) -> (2154.5545, 190.9445)
  line L190 (2121.2805, 175.0695) -> (2121.2805, 189.4205)
  arc A160 (1168.7805, 189.4205) -> (1167.2565, 190.9445) centre (1167.2565, 189.4205) ccw
  arc A161 (2121.2805, 189.4205) -> (2119.7565, 190.9445) centre (2119.7565, 189.4205) ccw
  line L191 (2387.9805, 189.4205) -> (2387.9805, 181.4195)
  line L192 (406.7805, 244.9195) -> (406.7805, 236.9185)
  arc A162 (1163.9545, 190.9445) -> (1162.4305, 189.4205) centre (1163.9545, 189.4205) ccw
  line L193 (2143.5055, 165.5445) -> (2130.8055, 165.5445)
  circle A163 centre (651.2555, 175.0695) radius 4.3815
  line L194 (1397.3805, 181.4195) -> (1168.7805, 181.4195)
  line L195 (2159.3805, 181.4195) -> (2159.3805, 189.4205)
  line L196 (2114.9305, 189.4205) -> (2114.9305, 181.4195)
  arc A164 (2387.9805, 236.9185) -> (2389.5045, 235.3945) centre (2389.5045, 236.9185) ccw
  line L197 (1124.3305, 181.4195) -> (946.5305, 181.4195)
  arc A165 (2121.2805, 175.0695) -> (2130.8055, 165.5445) centre (2130.8055, 175.0695) ccw
  arc A166 (2130.8055, 260.7945) -> (2121.2805, 251.2695) centre (2130.8055, 251.2695) ccw
  line L198 (1168.7805, 244.9195) -> (1397.3805, 244.9195)
  line L199 (1937.1305, 244.9195) -> (2114.9305, 244.9195)
  line L200 (902.0805, 181.4195) -> (673.4805, 181.4195)
  line L201 (2387.9805, 244.9195) -> (2387.9805, 236.9185)
  arc A167 (1152.9055, 165.5445) -> (1162.4305, 175.0695) centre (1152.9055, 175.0695) ccw
  arc A168 (2153.0305, 236.9185) -> (2154.5545, 235.3945) centre (2154.5545, 236.9185) ccw
  line L202 (2114.9305, 244.9195) -> (2114.9305, 236.9185)
  line L203 (2116.4545, 235.3945) -> (2119.7565, 235.3945)
  circle A169 centre (2137.1555, 175.0695) radius 4.3815
  line L204 (2153.0305, 251.2695) -> (2153.0305, 236.9185)
  line L205 (673.4805, 244.9195) -> (902.0805, 244.9195)
  line L206 (2114.9305, 181.4195) -> (1937.1305, 181.4195)
  line L207 (178.1805, 244.9195) -> (406.7805, 244.9195)
  arc A170 (1167.2565, 235.3945) -> (1168.7805, 236.9185) centre (1167.2565, 236.9185) ccw
  arc A171 (2153.0305, 251.2695) -> (2143.5055, 260.7945) centre (2143.5055, 251.2695) ccw
  arc A172 (2114.9305, 236.9185) -> (2116.4545, 235.3945) centre (2116.4545, 236.9185) ccw
  line L208 (1168.7805, 236.9185) -> (1168.7805, 244.9195)
  arc A173 (1162.4305, 251.2695) -> (1152.9055, 260.7945) centre (1152.9055, 251.2695) ccw
  line L209 (946.5305, 244.9195) -> (1124.3305, 244.9195)
  arc A174 (2116.4545, 190.9445) -> (2114.9305, 189.4205) centre (2116.4545, 189.4205) ccw
  arc A175 (1162.4305, 236.9185) -> (1163.9545, 235.3945) centre (1163.9545, 236.9185) ccw
  arc A176 (2389.5045, 190.9445) -> (2387.9805, 189.4205) centre (2389.5045, 189.4205) ccw
  line L210 (2159.3805, 244.9195) -> (2387.9805, 244.9195)
  line L211 (1162.4305, 189.4205) -> (1162.4305, 175.0695)
  line L212 (1168.7805, 181.4195) -> (1168.7805, 189.4205)
  line L213 (633.8565, 190.9445) -> (630.5545, 190.9445)
  line L214 (2130.8055, 260.7945) -> (2143.5055, 260.7945)
  arc A177 (667.1305, 236.9185) -> (668.6545, 235.3945) centre (668.6545, 236.9185) ccw
  arc A178 (1130.6805, 189.4205) -> (1129.1565, 190.9445) centre (1129.1565, 189.4205) ccw
  line L215 (2392.8065, 190.9445) -> (2389.5045, 190.9445)
  circle A179 centre (1146.5555, 251.2695) radius 4.3815
  line L216 (1124.3305, 189.4205) -> (1124.3305, 181.4195)
  arc A180 (2430.9065, 235.3945) -> (2432.4305, 236.9185) centre (2430.9065, 236.9185) ccw
  arc A181 (668.6545, 190.9445) -> (667.1305, 189.4205) centre (668.6545, 189.4205) ccw
  arc A182 (2157.8565, 235.3945) -> (2159.3805, 236.9185) centre (2157.8565, 236.9185) ccw
  arc A183 (657.6055, 165.5445) -> (667.1305, 175.0695) centre (657.6055, 175.0695) ccw
  arc A184 (673.4805, 189.4205) -> (671.9565, 190.9445) centre (671.9565, 189.4205) ccw
  line L217 (2121.2805, 236.9185) -> (2121.2805, 251.2695)
  arc A185 (671.9565, 235.3945) -> (673.4805, 236.9185) centre (671.9565, 236.9185) ccw
  line L218 (1124.3305, 244.9195) -> (1124.3305, 236.9185)
  line L219 (2389.5045, 235.3945) -> (2392.8065, 235.3945)
  arc A186 (1129.1565, 235.3945) -> (1130.6805, 236.9185) centre (1129.1565, 236.9185) ccw
  circle A187 centre (1146.5555, 175.0695) radius 4.3815
  line L220 (1125.8545, 235.3945) -> (1129.1565, 235.3945)
  arc A188 (2426.0805, 236.9185) -> (2427.6045, 235.3945) centre (2427.6045, 236.9185) ccw
  line L221 (635.3805, 175.0695) -> (635.3805, 189.4205)
  line L222 (673.4805, 181.4195) -> (673.4805, 189.4205)
  circle A189 centre (651.2555, 251.2695) radius 4.3815
  arc A190 (2416.5555, 165.5445) -> (2426.0805, 175.0695) centre (2416.5555, 175.0695) ccw
  line L223 (657.6055, 165.5445) -> (644.9055, 165.5445)
  arc A191 (644.9055, 260.7945) -> (635.3805, 251.2695) centre (644.9055, 251.2695) ccw
  line L224 (2430.9065, 190.9445) -> (2427.6045, 190.9445)
  arc A192 (635.3805, 175.0695) -> (644.9055, 165.5445) centre (644.9055, 175.0695) ccw
  arc A193 (1125.8545, 190.9445) -> (1124.3305, 189.4205) centre (1125.8545, 189.4205) ccw
  arc A194 (2154.5545, 190.9445) -> (2153.0305, 189.4205) centre (2154.5545, 189.4205) ccw
  line L225 (2119.7565, 190.9445) -> (2116.4545, 190.9445)
  line L226 (671.9565, 190.9445) -> (668.6545, 190.9445)
  arc A195 (2427.6045, 190.9445) -> (2426.0805, 189.4205) centre (2427.6045, 189.4205) ccw
  line L227 (2416.5555, 165.5445) -> (2403.8555, 165.5445)
  line L228 (1130.6805, 175.0695) -> (1130.6805, 189.4205)
  line L229 (1129.1565, 190.9445) -> (1125.8545, 190.9445)
  arc A196 (2394.3305, 189.4205) -> (2392.8065, 190.9445) centre (2392.8065, 189.4205) ccw
  line L230 (2427.6045, 235.3945) -> (2430.9065, 235.3945)
  arc A197 (635.3805, 189.4205) -> (633.8565, 190.9445) centre (633.8565, 189.4205) ccw
  line L231 (668.6545, 235.3945) -> (671.9565, 235.3945)
  line L232 (2153.0305, 189.4205) -> (2153.0305, 175.0695)
  line L233 (2432.4305, 244.9195) -> (2521.3305, 244.9195)
  line L234 (2521.3305, 181.4195) -> (2432.4305, 181.4195)
  line L235 (630.5545, 235.3945) -> (633.8565, 235.3945)
  arc A198 (1124.3305, 236.9185) -> (1125.8545, 235.3945) centre (1125.8545, 236.9185) ccw
  line L236 (1130.6805, 236.9185) -> (1130.6805, 251.2695)
  line L237 (644.9055, 260.7945) -> (657.6055, 260.7945)
  line L238 (2159.3805, 236.9185) -> (2159.3805, 244.9195)
  circle A199 centre (2410.2055, 175.0695) radius 4.3815
  arc A200 (667.1305, 251.2695) -> (657.6055, 260.7945) centre (657.6055, 251.2695) ccw
  line L239 (2394.3305, 236.9185) -> (2394.3305, 251.2695)
  arc A201 (2426.0805, 251.2695) -> (2416.5555, 260.7945) centre (2416.5555, 251.2695) ccw
  arc A202 (1140.2055, 260.7945) -> (1130.6805, 251.2695) centre (1140.2055, 251.2695) ccw
  arc A203 (2392.8065, 235.3945) -> (2394.3305, 236.9185) centre (2392.8065, 236.9185) ccw
  arc A204 (2403.8555, 260.7945) -> (2394.3305, 251.2695) centre (2403.8555, 251.2695) ccw
  line L240 (2426.0805, 189.4205) -> (2426.0805, 175.0695)
  line L241 (667.1305, 189.4205) -> (667.1305, 175.0695)
  arc A205 (2432.4305, 189.4205) -> (2430.9065, 190.9445) centre (2430.9065, 189.4205) ccw
  line L242 (2394.3305, 175.0695) -> (2394.3305, 189.4205)
  arc A206 (1130.6805, 175.0695) -> (1140.2055, 165.5445) centre (1140.2055, 175.0695) ccw
  arc A207 (1664.0805, 189.4205) -> (1662.5565, 190.9445) centre (1662.5565, 189.4205) ccw
  line L243 (1659.2545, 235.3945) -> (1662.5565, 235.3945)
  arc A208 (1657.7305, 251.2695) -> (1648.2055, 260.7945) centre (1648.2055, 251.2695) ccw
  line L244 (1664.0805, 236.9185) -> (1664.0805, 244.9195)
  line L245 (1932.3045, 235.3945) -> (1935.6065, 235.3945)
  arc A209 (1657.7305, 236.9185) -> (1659.2545, 235.3945) centre (1659.2545, 236.9185) ccw
  arc A210 (1662.5565, 235.3945) -> (1664.0805, 236.9185) centre (1662.5565, 236.9185) ccw
  arc A211 (1659.2545, 190.9445) -> (1657.7305, 189.4205) centre (1659.2545, 189.4205) ccw
  line L246 (1657.7305, 251.2695) -> (1657.7305, 236.9185)
  line L247 (1930.7805, 251.2695) -> (1930.7805, 236.9185)
  line L248 (1662.5565, 190.9445) -> (1659.2545, 190.9445)
  line L249 (1930.7805, 189.4205) -> (1930.7805, 175.0695)
  arc A212 (1648.2055, 165.5445) -> (1657.7305, 175.0695) centre (1648.2055, 175.0695) ccw
  arc A213 (1908.5555, 260.7945) -> (1899.0305, 251.2695) centre (1908.5555, 251.2695) ccw
  line L250 (1897.5065, 190.9445) -> (1894.2045, 190.9445)
  line L251 (1908.5555, 260.7945) -> (1921.2555, 260.7945)
  line L252 (1899.0305, 236.9185) -> (1899.0305, 251.2695)
  arc A214 (1921.2555, 165.5445) -> (1930.7805, 175.0695) centre (1921.2555, 175.0695) ccw
  circle A215 centre (1914.9055, 175.0695) radius 4.3815
  line L253 (1894.2045, 235.3945) -> (1897.5065, 235.3945)
  arc A216 (1935.6065, 235.3945) -> (1937.1305, 236.9185) centre (1935.6065, 236.9185) ccw
  line L254 (1937.1305, 181.4195) -> (1937.1305, 189.4205)
  arc A217 (1897.5065, 235.3945) -> (1899.0305, 236.9185) centre (1897.5065, 236.9185) ccw
  arc A218 (1932.3045, 190.9445) -> (1930.7805, 189.4205) centre (1932.3045, 189.4205) ccw
  arc A219 (1899.0305, 189.4205) -> (1897.5065, 190.9445) centre (1897.5065, 189.4205) ccw
  arc A220 (1937.1305, 189.4205) -> (1935.6065, 190.9445) centre (1935.6065, 189.4205) ccw
  line L255 (1921.2555, 165.5445) -> (1908.5555, 165.5445)
  line L256 (1899.0305, 175.0695) -> (1899.0305, 189.4205)
  line L257 (1935.6065, 190.9445) -> (1932.3045, 190.9445)
  line L258 (1937.1305, 236.9185) -> (1937.1305, 244.9195)
  arc A221 (1930.7805, 236.9185) -> (1932.3045, 235.3945) centre (1932.3045, 236.9185) ccw
  circle A222 centre (1914.9055, 251.2695) radius 4.3815
  arc A223 (1930.7805, 251.2695) -> (1921.2555, 260.7945) centre (1921.2555, 251.2695) ccw
  arc A224 (1899.0305, 175.0695) -> (1908.5555, 165.5445) centre (1908.5555, 175.0695) ccw
  line L259 (1635.5055, 260.7945) -> (1648.2055, 260.7945)
  line L260 (1403.7305, 236.9185) -> (1403.7305, 251.2695)
  line L261 (1441.8305, 181.4195) -> (1441.8305, 189.4205)
  line L262 (1441.8305, 244.9195) -> (1619.6305, 244.9195)
  line L263 (1619.6305, 181.4195) -> (1441.8305, 181.4195)
  line L264 (1648.2055, 165.5445) -> (1635.5055, 165.5445)
  line L265 (1398.9045, 235.3945) -> (1402.2065, 235.3945)
  arc A225 (1440.3065, 235.3945) -> (1441.8305, 236.9185) centre (1440.3065, 236.9185) ccw
  line L266 (1441.8305, 236.9185) -> (1441.8305, 244.9195)
  arc A226 (1441.8305, 189.4205) -> (1440.3065, 190.9445) centre (1440.3065, 189.4205) ccw
  line L267 (1403.7305, 175.0695) -> (1403.7305, 189.4205)
  line L268 (1413.2555, 260.7945) -> (1425.9555, 260.7945)
  line L269 (1397.3805, 244.9195) -> (1397.3805, 236.9185)
  arc A227 (1398.9045, 190.9445) -> (1397.3805, 189.4205) centre (1398.9045, 189.4205) ccw
  arc A228 (1403.7305, 175.0695) -> (1413.2555, 165.5445) centre (1413.2555, 175.0695) ccw
  arc A229 (1435.4805, 251.2695) -> (1425.9555, 260.7945) centre (1425.9555, 251.2695) ccw
  arc A230 (1425.9555, 165.5445) -> (1435.4805, 175.0695) centre (1425.9555, 175.0695) ccw
  line L270 (1425.9555, 165.5445) -> (1413.2555, 165.5445)
  line L271 (1435.4805, 189.4205) -> (1435.4805, 175.0695)
  arc A231 (1435.4805, 236.9185) -> (1437.0045, 235.3945) centre (1437.0045, 236.9185) ccw
  arc A232 (1413.2555, 260.7945) -> (1403.7305, 251.2695) centre (1413.2555, 251.2695) ccw
  line L272 (1402.2065, 190.9445) -> (1398.9045, 190.9445)
  arc A233 (1397.3805, 236.9185) -> (1398.9045, 235.3945) centre (1398.9045, 236.9185) ccw
  arc A234 (1437.0045, 190.9445) -> (1435.4805, 189.4205) centre (1437.0045, 189.4205) ccw
  line L273 (1440.3065, 190.9445) -> (1437.0045, 190.9445)
  line L274 (1397.3805, 189.4205) -> (1397.3805, 181.4195)
  line L275 (1435.4805, 251.2695) -> (1435.4805, 236.9185)
  line L276 (1437.0045, 235.3945) -> (1440.3065, 235.3945)
  arc A235 (1403.7305, 189.4205) -> (1402.2065, 190.9445) centre (1402.2065, 189.4205) ccw
  circle A236 centre (1419.6055, 175.0695) radius 4.3815
  circle A237 centre (1419.6055, 251.2695) radius 4.3815
  line L277 (1892.6805, 181.4195) -> (1664.0805, 181.4195)
  line L278 (1892.6805, 244.9195) -> (1892.6805, 236.9185)
  line L279 (1664.0805, 244.9195) -> (1892.6805, 244.9195)
  arc A238 (1625.9805, 189.4205) -> (1624.4565, 190.9445) centre (1624.4565, 189.4205) ccw
  line L280 (1624.4565, 190.9445) -> (1621.1545, 190.9445)
  line L281 (1892.6805, 189.4205) -> (1892.6805, 181.4195)
  arc A239 (1892.6805, 236.9185) -> (1894.2045, 235.3945) centre (1894.2045, 236.9185) ccw
  arc A240 (1894.2045, 190.9445) -> (1892.6805, 189.4205) centre (1894.2045, 189.4205) ccw
  line L282 (1657.7305, 189.4205) -> (1657.7305, 175.0695)
  line L283 (1664.0805, 181.4195) -> (1664.0805, 189.4205)
  arc A241 (1625.9805, 175.0695) -> (1635.5055, 165.5445) centre (1635.5055, 175.0695) ccw
  line L284 (1619.6305, 244.9195) -> (1619.6305, 236.9185)
  line L285 (1625.9805, 236.9185) -> (1625.9805, 251.2695)
  circle A242 centre (1641.8555, 251.2695) radius 4.3815
  line L286 (1625.9805, 175.0695) -> (1625.9805, 189.4205)
  line L287 (1621.1545, 235.3945) -> (1624.4565, 235.3945)
  line L288 (1619.6305, 189.4205) -> (1619.6305, 181.4195)
  circle A243 centre (1641.8555, 175.0695) radius 4.3815
  arc A244 (1635.5055, 260.7945) -> (1625.9805, 251.2695) centre (1635.5055, 251.2695) ccw
  arc A245 (1402.2065, 235.3945) -> (1403.7305, 236.9185) centre (1402.2065, 236.9185) ccw
  arc A246 (1619.6305, 236.9185) -> (1621.1545, 235.3945) centre (1621.1545, 236.9185) ccw
  arc A247 (1624.4565, 235.3945) -> (1625.9805, 236.9185) centre (1624.4565, 236.9185) ccw
  arc A248 (1621.1545, 190.9445) -> (1619.6305, 189.4205) centre (1621.1545, 189.4205) ccw
  arc A249 (138.5565, 235.3945) -> (140.0805, 236.9185) centre (138.5565, 236.9185) ccw
  arc A250 (140.0805, 175.0695) -> (149.6055, 165.5445) centre (149.6055, 175.0695) ccw
  arc A251 (446.4045, 190.9445) -> (444.8805, 189.4205) centre (446.4045, 189.4205) ccw
  line L289 (451.2305, 236.9185) -> (451.2305, 244.9195)
  circle A252 centre (155.9555, 175.0695) radius 4.3815
  arc A253 (422.6555, 260.7945) -> (413.1305, 251.2695) centre (422.6555, 251.2695) ccw
  line L290 (162.3055, 165.5445) -> (149.6055, 165.5445)
  line L291 (446.4045, 235.3945) -> (449.7065, 235.3945)
  line L292 (173.3545, 235.3945) -> (176.6565, 235.3945)
  line L293 (149.6055, 260.7945) -> (162.3055, 260.7945)
  line L294 (135.2545, 235.3945) -> (138.5565, 235.3945)
  line L295 (133.7305, 189.4205) -> (133.7305, 181.4195)
  line L296 (178.1805, 181.4195) -> (178.1805, 189.4205)
  line L297 (178.1805, 236.9185) -> (178.1805, 244.9195)
  line L298 (413.1305, 175.0695) -> (413.1305, 189.4205)
  circle A254 centre (429.0055, 175.0695) radius 4.3815
  line L299 (413.1305, 236.9185) -> (413.1305, 251.2695)
  arc A255 (176.6565, 235.3945) -> (178.1805, 236.9185) centre (176.6565, 236.9185) ccw
  line L300 (176.6565, 190.9445) -> (173.3545, 190.9445)